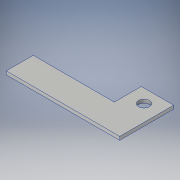
# Autodesk Inventor part: Y-axis Carriage Flag
Saved by Autodesk Inventor 2018 (Build 220112000, 112)
## iProperties
Created: 2013-10-27
Part Number: Y-axis Carriage Flag
Material: Aluminum 6061
Document SubType Name: Modeling
Designer: Gabriel Smolnycki
Mass: 2.84814 g
Surface Area: 13.28 cm^2
Volume: 1.05487 cm^3
Density: 2.7 g/cm^3
Appearance: Aluminum - Flat
Sending System: SolidWorks 2017
Last Author: Gabriel Smolnycki
Last Saved: 2017-09-14
Author: Gabriel Smolnycki
Autodesk Inventor part; units mm, degrees
ref_plane "YZ Plane" through (0, 0, 0) normal (1, 0, 0) x (0, 1, 0)
ref_plane "XZ Plane" through (0, 0, 0) normal (0, 1, 0) x (-1, 0, 0)
ref_plane "XY Plane" through (0, 0, 0) normal (0, 0, 1) x (1, 0, 0)
sketch "Sketch1" plane through (0, 0, 0) normal (0, 1, 0) x (-1, 0, 0)
  line L0 (0, 0) -> (0, -20)
  line L1 (42, 0) -> (0, 0)
  line L2 (42, -10) -> (42, 0)
  line L3 (12, -10) -> (42, -10)
  line L4 (12, -20) -> (12, -10)
  line L5 (0, -20) -> (12, -20)
  constraints: 12 end point, 3 horizontal, 3 vertical, 1 parallel
extrude "Extrusion1" add sketch "Sketch1" along normal blind 1.27
sketch "Sketch2" plane through (0, 1.27, 0) normal (0, 1, 0) x (1, 0, 0)
  point P0 (-6, 15)
hole "Hole1" at (-6, 1.27, -15) direction (0, -1, 0) diameter 4 depth 1.27 tip angle 118
body "Solid3"
